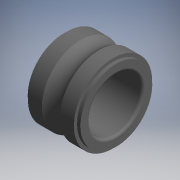
# Autodesk Inventor part: F606ZZ Inner Ring
Saved by Autodesk Inventor 2017.3 (Build 213256000, 256)
## iProperties
Part Number: F606ZZ Inner Ring
Material: Generic
Catalog Web Link: www.cadenas.de
Description: shielded_type_zz_zzs_IR-
Vendor: NSK_RB
Document SubType Name: Modeling
Designer: partserver
Manufacturer: NSK_RB
Mass: 0.183587 g
Surface Area: 3.44472 cm^2
Volume: 0.183587 cm^3
Density: 1 g/cm^3
Appearance: PSOLRGB-128-128-128
Category: PARTsolutions
Company: NSK_RB
Title: F606ZZ Inner Ring
Author: Cadenas PARTsolutions
PSOL_IDENT_0: {$CADENAS_DATA\23d-libs\nsk_rb\roller_bearings\deep_groove_bb\exstra_small_miniatur_bb\metric_design
PSOL_IDENT_1: _with_flange\shielded_type_zz_zzs_ir_1.prj},192 {VTYP=3D},{NB=F606ZZ Inner Ring},{LINA=F606ZZ Inner
PSOL_IDENT_2: Ring},{NN=shielded_type_zz_zzs_IR},{DATE=10.04.2020 04:57:40},{GEOMDATE=04.01.2008 00:00:00},{VERSIO
PSOL_IDENT_3: N=},{LINEID=540},{WBVAR=},{WBNUMERIC=}  {NB=F606ZZ Inner Ring},{LINA=F606ZZ Inner Ring},{KT=DUMMY},{
PSOL_IDENT_4: IDNR=},{STAN=},{ORDER=F606ZZ},{SD=6.0},{X=6.0},{D=17},{DD=17},{DD1=0.0},{D2=19.0},{DD2=19.0},{B=0.0}
PSOL_IDENT_5: ,{B1=6.0},{CC1=0.0},{C2=1.2},{CC2=1.2},{R=0.00},{R1=0.30},{DI1=8.92},{DI2=8.20},{SDE1=13.75},{SDE2=1
PSOL_IDENT_6: 4.80},{CR1=2260},{COR1=835},{CR2=231},{COR2=85.0},{LG=38000},{LO=45000},{DA=0.0},{DB=8.2},{RA=0.00},
PSOL_IDENT_7: {RB=0.30},{MASS=6.61},{SC=1},{N=8}
NB: F606ZZ Inner Ring
NN: shielded_type_zz_zzs_IR
NBSYN: $ORDER. Inner Ring
LINA: F606ZZ Inner Ring
CATALOG: NSK Rolling Bearing
ORDER: F606ZZ
SD: 6
X: 6
D: 17
DD: 17
DD1: 0
D2: 19
DD2: 19
B: 0
B1: 6
CC1: 0
C2: 1.2
CC2: 1.2
R: 0
R1: 0.3
DI1: 8.92
DI2: 8.2
SDE1: 13.75
SDE2: 14.8
CR1: 2260
COR1: 835
CR2: 231
COR2: 85
LG: 38000
LO: 45000
DA: 0
DB: 8.2
RA: 0
RB: 0.3
MASS: 6.61
SC: 1
SUPPLIER: NSK_RB
ARTICLENO: F606ZZ Inner Ring
BOMINFO: F606ZZ Inner Ring
CREATOR: CADENAS GmbH
Autodesk Inventor part; units mm, degrees
ref_plane "YZ Plane" through (0, 0, 0) normal (1, 0, 0) x (0, 1, 0)
ref_plane "XZ Plane" through (0, 0, 0) normal (0, 1, 0) x (-1, 0, 0)
ref_plane "XY Plane" through (0, 0, 0) normal (0, 0, 1) x (1, 0, 0)
sketch "Sketch_2" plane through (0, 0, 0) normal (0, 0, 1) x (1, 0, 0)
  line L0 (6, 0) -> (0, 0)
  arc A0 (0, 3.3) -> (0.3, 3) centre (0.3, 3.3) ccw
  line L1 (0.3, 3) -> (5.7, 3)
  arc A1 (5.7, 3) -> (6, 3.3) centre (5.7, 3.3) ccw
  line L2 (6, 3.3) -> (6, 4.1)
  line L3 (6, 4.1) -> (5.625, 4.1)
  line L4 (5.625, 4.1) -> (5.625, 4.46)
  line L5 (5.625, 4.46) -> (4.0288, 4.46)
  arc A2 (1.9712, 4.46) -> (4.0288, 4.46) centre (3, 5.75) ccw
  line L6 (1.9712, 4.46) -> (0.375, 4.46)
  line L7 (0.375, 4.46) -> (0.375, 4.1)
  line L8 (0.375, 4.1) -> (0, 4.1)
  line L9 (0, 4.1) -> (0, 3.3)
  constraints: 20 end point, 6 point on circle, 3 centre point
revolve "Revolution1" add sketch "Sketch_2" angle 360 about axis through (6, 0, 0) along (1, 0, 0)
ref_plane "ip_st_1_1_XY" through (3, 5.75, 0) normal (1, 0, 0) x (0, 0, -1)
ref_plane "ip_st_1_1_YZ" through (3, 5.75, 0) normal (0, 0, -1) x (0, 1, 0)
ref_plane "ip_st_1_1_ZX" through (3, 5.75, 0) normal (0, 1, 0) x (1, 0, 0)
ref_plane "ip_st_1_2_XY" through (3, 4.0659, 4.0659) normal (1, 0, 0) x (0, 0, -1)
ref_plane "ip_st_1_2_YZ" through (3, 4.0659, 4.0659) normal (0, 0, -1) x (0, 1, 0)
ref_plane "ip_st_1_2_ZX" through (3, 4.0659, 4.0659) normal (0, 1, 0) x (1, 0, 0)
ref_plane "ip_st_1_3_XY" through (3, 0, 5.75) normal (1, 0, 0) x (0, 0, -1)
ref_plane "ip_st_1_3_YZ" through (3, 0, 5.75) normal (0, 0, -1) x (0, 1, 0)
ref_plane "ip_st_1_3_ZX" through (3, 0, 5.75) normal (0, 1, 0) x (1, 0, 0)
ref_plane "ip_st_1_4_XY" through (3, -4.0659, 4.0659) normal (1, 0, 0) x (0, 0, -1)
ref_plane "ip_st_1_4_YZ" through (3, -4.0659, 4.0659) normal (0, 0, -1) x (0, 1, 0)
ref_plane "ip_st_1_4_ZX" through (3, -4.0659, 4.0659) normal (0, 1, 0) x (1, 0, 0)
ref_plane "ip_st_1_5_XY" through (3, -5.75, 0) normal (1, 0, 0) x (0, 0, -1)
ref_plane "ip_st_1_5_YZ" through (3, -5.75, 0) normal (0, 0, -1) x (0, 1, 0)
ref_plane "ip_st_1_5_ZX" through (3, -5.75, 0) normal (0, 1, 0) x (1, 0, 0)
ref_plane "ip_st_1_6_XY" through (3, -4.0659, -4.0659) normal (1, 0, 0) x (0, 0, -1)
ref_plane "ip_st_1_6_YZ" through (3, -4.0659, -4.0659) normal (0, 0, -1) x (0, 1, 0)
ref_plane "ip_st_1_6_ZX" through (3, -4.0659, -4.0659) normal (0, 1, 0) x (1, 0, 0)
ref_plane "ip_st_1_7_XY" through (3, 0, -5.75) normal (1, 0, 0) x (0, 0, -1)
ref_plane "ip_st_1_7_YZ" through (3, 0, -5.75) normal (0, 0, -1) x (0, 1, 0)
ref_plane "ip_st_1_7_ZX" through (3, 0, -5.75) normal (0, 1, 0) x (1, 0, 0)
ref_plane "ip_st_1_8_XY" through (3, 4.0659, -4.0659) normal (1, 0, 0) x (0, 0, -1)
ref_plane "ip_st_1_8_YZ" through (3, 4.0659, -4.0659) normal (0, 0, -1) x (0, 1, 0)
ref_plane "ip_st_1_8_ZX" through (3, 4.0659, -4.0659) normal (0, 1, 0) x (1, 0, 0)
ref_plane "ip_st_1a_XY" through (0, 0, 0) normal (1, 0, 0) x (0, 0, -1)
ref_plane "ip_st_1a_YZ" through (0, 0, 0) normal (0, 0, -1) x (0, 1, 0)
ref_plane "ip_st_1a_ZX" through (0, 0, 0) normal (0, 1, 0) x (1, 0, 0)
ref_plane "ip_st_2a_XY" through (0.375, 0, 0) normal (1, 0, 0) x (0, 0, -1)
ref_plane "ip_st_2a_YZ" through (0.375, 0, 0) normal (0, 0, -1) x (0, 1, 0)
ref_plane "ip_st_2a_ZX" through (0.375, 0, 0) normal (0, 1, 0) x (1, 0, 0)
body "Solid1"
